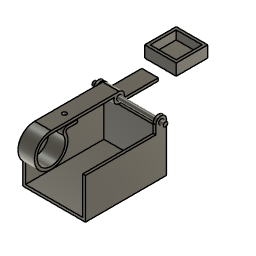
Card Holder v15 (Autodesk Fusion 360 design; units mm, degrees)
Autodesk Fusion 360 part; units mm, degrees
note: some values were not read from the file. Set by a fixed rule: which face or edge a step refers to.
sketch "Sketch1" plane through (0, 0, 0) normal (0, 0, 1) x (1, 0, 0)
  line L0 (0, 0) -> (66, 0)
  line L1 (66, 0) -> (66, 90.5)
  line L2 (66, 90.5) -> (0, 90.5)
  line L3 (0, 90.5) -> (0, 0)
  dimension "d12" = 66
  dimension "d13" = 90.5
  constraint horizontal L0
  constraint vertical L1
  constraint horizontal L2
  constraint vertical L3
  constraint coincident L0.start L3.end
  measures "d12" distance of L0.start L0.end
  measures "d13" distance of L0.end L1.end
extrude "Extrude1" add sketch "Sketch1" along normal blind 43.5 makes body 1
shell "Shell1" thickness 3.2 outward yes removed faces 2 at (44, 0, 14.5) at (22, 60.3333, 43.5) on bodies 1
sketch "Sketch2" plane through (-3.2, 0, 0) normal (-1, 0, 0) x (0, -1, 0)
  line L0 (-93.7, -3.2) -> (0, -3.2)
  line L1 (0, -3.2) -> (0, 43.5)
  line L2 (0, 43.5) -> (-93.7, 43.5)
  line L3 (-93.7, 43.5) -> (-93.7, -3.2)
  circle A0 centre (-87.6, 53.5) radius 2.5
  circle A1 centre (-87.6, 53.5) radius 2.9
  circle A2 centre (-87.6, 53.5) radius 6.1
  line L4 (-93.7, 53.5) -> (-93.7, 43.5)
  line L5 (-81.5, 53.5) -> (-81.5, 43.5)
  dimension "d17" = 5
  dimension "d18" = 0.4
  dimension "d19" = 3.2
  dimension "d20" = 10
  constraint concentric A0 A1
  constraint concentric A0 A2
  constraint coincident A2 L4.start
  constraint tangent A2 L4
  constraint coincident A2 L5.start
  constraint tangent A2 L5
  constraint vertical L4
  constraint vertical L5
  constraint horizontal L2.end L5.end
  constraint coincident L2.end L3.start
  measures "d17" diameter of A0
  measures "d18" distance of A0 A1
  measures "d19" distance of A1 A2
  measures "d20" distance of L2 A0.centre
extrude "Extrude2" add sketch "Sketch2" against normal up to surface (3.2 mm away) contours L2 A2 L4 L5 | A2 bodies 1
extrude "Extrude3" add sketch "Sketch2" against normal up to surface (3.2 mm away) from surface at -69.2 contours L2 A2 L4 L5 | A2 bodies 1
ref_plane "WorkPlane3" through (74.2, 46.85, 28.2) normal (1, 0, 0) x (0, 1, 0)
extrude "Extrude4" add sketch "Sketch2" along normal blind 5 and the other way up to surface (77.4 mm away) separate body contours A0 makes body 2
ref_plane "WorkPlane1" through (-3.2, 46.85, 28.2) normal (-1, 0, 0) x (0, -1, 0)
sketch "Sketch4" plane through (-3.2, 0, 0) normal (-1, 0, 0) x (0, -1, 0)
  circle A0 centre (-87.6, 53.5) radius 2.5
  circle A1 centre (-87.6, 53.5) radius 2.9
  circle A2 centre (-87.6, 53.5) radius 6.1
  line L0 (-87.6, 59.6) -> (2.9, 59.6)
  line L1 (2.9, 59.6) -> (2.9, 56.4)
  line L2 (2.9, 56.4) -> (-87.6, 56.4)
  line L3 (-32.7, 110) -> (-32.7, 124.9)
  line L4 (-32.7, 124.9) -> (-12.7, 124.9)
  line L5 (-12.7, 124.9) -> (-12.7, 110)
  line L6 (-32.7, 110) -> (-35.9, 110)
  line L7 (-35.9, 110) -> (-35.9, 128.1)
  line L8 (-35.9, 128.1) -> (-9.5, 128.1)
  line L9 (-9.5, 128.1) -> (-9.5, 110)
  line L10 (-12.7, 110) -> (-9.5, 110)
  line L11 (-87.6, 56.4) -> (-87.6, 59.6)
  circle A3 centre (-9, 40.225) radius 16.175
  circle A4 centre (-9, 40.225) radius 19.375
  line L12 (0, -3.2) -> (0, 43.5)
  line L13 (-39.575, 55.6) -> (-28.375, 55.6)
  line L14 (-28.375, 55.6) -> (-28.375, 52.4)
  line L15 (-28.375, 52.4) -> (-39.575, 52.4)
  line L16 (-39.575, 52.4) -> (-39.575, 55.6)
  circle A5 centre (-28.375, 50.0509) radius 2.3491
  circle A6 centre (-28.375, 50.0509) radius 5.5491
  line L17 (-132.85, 50.6) -> (-87.6, 50.6)
  line L18 (-87.6, 50.6) -> (-87.6, 47.4)
  line L19 (-87.6, 47.4) -> (-132.85, 47.4)
  line L20 (-132.85, 47.4) -> (-132.85, 50.6)
  dimension "d34" = 5.8
  dimension "d35" = 3.2
  dimension "d36" = 3.2
  dimension "d37" = 90.5
  dimension "d38" = 3.2
  dimension "d39" = 3.2
  dimension "d40" = 3.2
  dimension "d41" = 14.9
  dimension "d42" = 20
  dimension "d43" = 50.4
  dimension "d44" = 12.4
  dimension "d84" = 32.35
  dimension "d85" = 3.2
  dimension "d87" = 9
  dimension "d88" = 3.2
  dimension "d89" = 0.8
  dimension "d90" = 11.2
  dimension "d97" = 45.25
  dimension "d98" = 3.2
  constraint concentric A0 A1
  constraint concentric A0 A2
  constraint horizontal L0
  constraint vertical L1
  constraint horizontal L2
  constraint coincident A2 L0.start
  constraint vertical A0.centre L0.start
  constraint vertical L3
  constraint perpendicular L3 L4
  constraint perpendicular L4 L5
  constraint perpendicular L3 L6
  constraint perpendicular L6 L7
  constraint perpendicular L7 L8
  constraint perpendicular L8 L9
  constraint perpendicular L9 L10
  constraint horizontal L6.end L9.end
  constraint vertical L11
  constraint coincident L2.end L11.start
  constraint concentric A3 A4
  constraint tangent L0 A4
  constraint horizontal L13
  constraint vertical L14
  constraint horizontal L15
  constraint vertical L16
  constraint tangent A4 L14
  constraint concentric A5 A6
  constraint tangent A3 A6
  constraint tangent A4 A5
  constraint tangent L13 A6
  constraint coincident L14.end A5
  constraint horizontal L17
  constraint vertical L18
  constraint horizontal L19
  constraint vertical L20
  constraint collinear L11 L18
  constraint coincident A1 L17.end
  measures "d34" diameter of A1
  measures "d35" distance of A1 A2
  measures "d36" distance of L0.end L1.end
  measures "d37" distance of L0.start L0.end
  measures "d38" distance of L3.start L6.end
  measures "d39" distance of L5.end L9.end
  measures "d40" distance of L4 L8
  measures "d41" distance of L3.start L3.end
  measures "d42" distance of L3.end L4.end
  measures "d43" vertical distance of L0.end L9.end
  measures "d44" horizontal distance of L0.end L9.end
  measures "d84" diameter of A3
  measures "d85" distance of A3 A4
  measures "d87" distance of A3.centre L12
  measures "d88" distance of L13.start L15.end
  measures "d89" distance of L2 L13
  measures "d90" distance of L14.end L15.end
  measures "d97" distance of L18.end L19.end
  measures "d98" distance of L17.start L19.end
extrude "Extrude5" add sketch "Sketch4" against normal blind 19 from surface at -4.8 separate body contours A1 A2 L2 L18 | A2 L2 L11 | A1 A2 L11 L17 | A2 L17 L18 | A2 L0 L2 A4 | A2 L17 L19 L20 | L2 A4 | L2 A3 A4 L12 | A4 A6 | A4 L14 A5 A6 | A3 A4 L12 A6 | L13 L15 L16 A6 | L14 L15 A6 makes body 3
ref_plane "WorkPlane4" through (11.1, 48.3, 59.6) normal (0, 0, 1) x (0, -1, 0)
sketch "Sketch7" plane through (0, 0, 59.6) normal (0, 0, 1) x (1, 0, 0)
  line L0 (1.6, 39.575) -> (1.6, 28.375)
  line L1 (1.6, 28.375) -> (20.6, 28.375)
  line L2 (20.6, 28.375) -> (20.6, 39.575)
  line L3 (20.6, 39.575) -> (1.6, 39.575)
  circle A0 centre (11.1, 33.975) radius 2
  circle A1 centre (11.1, 33.975) radius 2.4
  point P0 (11.1, 39.575)
  dimension "d92" = 5.6
  dimension "d93" = 4
  dimension "d94" = 0.4
  constraint concentric A0 A1
  constraint midpoint L3 P0
  constraint vertical A0.centre P0
  measures "d92" distance of L3 A0.centre
  measures "d93" diameter of A0
  measures "d94" distance of A0 A1
extrude "Extrude10" cut sketch "Sketch7" against normal up to surface (7.2 mm away) contours A0 | A1 bodies 3
sketch "Sketch6" plane through (0, 0, 50.6) normal (0, 0, 1) x (-1, 0, 0)
  line L0 (-1.6, -87.6) -> (-1.6, -9)
  line L1 (-20.6, -9) -> (-20.6, -87.6)
  line L2 (3.9, -178.1) -> (-26.1, -178.1)
  line L3 (-26.1, -178.1) -> (-26.1, -148.1)
  line L4 (-26.1, -148.1) -> (3.9, -148.1)
  line L5 (3.9, -148.1) -> (3.9, -178.1)
  line L6 (7.1, -144.9) -> (7.1, -181.3)
  line L7 (7.1, -181.3) -> (-29.3, -181.3)
  line L8 (-29.3, -181.3) -> (-29.3, -144.9)
  line L9 (-29.3, -144.9) -> (7.1, -144.9)
  line L10 (-1.6, -9) -> (-20.6, -9)
  circle A0 centre (-11.1, -33.775) radius 2.4
  line L11 (-20.6, -87.6) -> (-1.6, -87.6)
  line L12 (-1.6, -132.85) -> (-1.6, -92.9666)
  line L13 (-1.6, -92.9666) -> (-20.6, -92.9666)
  line L14 (-20.6, -92.9666) -> (-20.6, -132.85)
  line L15 (-20.6, -132.85) -> (-1.6, -132.85)
  point P0 (-11.1, -178.1)
  point P1 (-11.1, -178.1)
  dimension "d76" = 30
  dimension "d77" = 30
  constraint horizontal L2
  constraint vertical L3
  constraint horizontal L4
  constraint vertical L5
  constraint midpoint L2 P1
  constraint coincident P1 P0
  measures "d76" distance of L2.start L2.end
  measures "d77" distance of L2.end L3.end
extrude "Extrude8" add sketch "Sketch6" along normal blind 3.2 separate body contours L2 L3 L4 L5 makes body 4
extrude "Extrude9" add sketch "Sketch6" along normal blind 13.2 contours L6 L7 L8 L9 bodies 4 3
ref_plane "WorkPlane2" through (11.1, 11.1, 110) normal (0, 0, -1) x (0, 1, 0)
sketch "Sketch5" plane through (0, 0, 110) normal (0, 0, -1) x (-1, 0, 0)
  circle A0 centre (-11.1, 41.5) radius 2
  circle A1 centre (-11.1, 41.5) radius 2.4
  line L0 (-1.6, 35.9) -> (-20.6, 35.9)
  circle A2 centre (-11.1, 3.9) radius 2
  circle A3 centre (-11.1, 3.9) radius 2.4
  line L1 (-1.6, 9.5) -> (-20.6, 9.5)
  line L2 (-1.6, 47.1) -> (-20.6, 47.1)
  line L3 (-20.6, 47.1) -> (-20.6, 35.9)
  line L4 (-20.6, 35.9) -> (-1.6, 35.9)
  line L5 (-1.6, 35.9) -> (-1.6, 47.1)
  line L6 (-1.6, -1.7) -> (-20.6, -1.7)
  line L7 (-20.6, -1.7) -> (-20.6, 9.5)
  line L8 (-20.6, 9.5) -> (-1.6, 9.5)
  line L9 (-1.6, 9.5) -> (-1.6, -1.7)
  point P0 (-11.1, 35.9)
  point P1 (-11.1, -1.7)
  point P2 (-11.1, 47.1)
  dimension "d49" = 4
  dimension "d51" = 0.4
  dimension "d53" = 4
  dimension "d55" = 0.4
  dimension "d67" = 5.6
  dimension "d68" = 5.6
  dimension "d70" = 5.6
  dimension "d71" = 5.6
  constraint concentric A0 A1
  constraint midpoint L0 P0
  constraint concentric A2 A3
  constraint vertical P0 A2.centre
  constraint horizontal L2
  constraint vertical L3
  constraint horizontal L4
  constraint vertical L5
  constraint coincident L0 L3.end
  constraint vertical L7
  constraint horizontal L8
  constraint vertical L9
  constraint coincident L1 L7.end
  constraint midpoint L6 P1
  constraint vertical A2.centre P1
  constraint horizontal L6
  constraint coincident L1.end L7.end
  constraint midpoint L2 P2
  constraint vertical A0.centre P2
  constraint coincident L0.start L4.end
  constraint vertical P0 A0.centre
  measures "d49" diameter of A0
  measures "d51" distance of A0 A1
  measures "d53" diameter of A2
  measures "d55" distance of A2 A3
  measures "d67" distance of A2.centre L8
  measures "d68" distance of A2.centre L6
  measures "d70" vertical distance of A0.centre P0
  measures "d71" distance of L2 A0.centre
extrude "Extrude6" [suppressed]
fillet "Fillet1" [suppressed]
extrude "Extrude7" [suppressed]
equation "CardWidth = 66 mm"
equation "CardHeight = 90.5 mm"
equation "CardDepth = 14.5 mm * 3"
equation "MotorHeight = 14.9 mm"
equation "MotorWidth = 20 mm"
equation "MotorPlatformDepth = 19 mm"
equation "Tolerance = 0.4 mm"
equation "RodDiameter = 5 mm"
equation "ScrewBigDiameter = 5.6 mm"
equation "ScrewSmallDiameter = 4 mm"
equation "WallThickness = 3.2 mm"
equation "d12 = CardWidth"
equation "d13 = CardHeight"
equation "d14 = CardDepth"
equation "d16 = WallThickness"
equation "d17 = RodDiameter"
equation "d18 = Tolerance"
equation "d19 = WallThickness"
equation "d34 = RodDiameter + 2 * Tolerance"
equation "d35 = WallThickness"
equation "d36 = WallThickness"
equation "d37 = CardHeight"
equation "d38 = WallThickness"
equation "d39 = WallThickness"
equation "d40 = WallThickness"
equation "d41 = MotorHeight"
equation "d42 = MotorWidth"
equation "d43 = Tolerance + 50 mm"
equation "d44 = 2 * WallThickness + ScrewSmallDiameter + 5 * Tolerance"
equation "d45 = -WallThickness - 4 * Tolerance"
equation "d46 = -MotorPlatformDepth"
equation "d49 = ScrewSmallDiameter"
equation "d51 = Tolerance"
equation "d53 = ScrewSmallDiameter"
equation "d55 = Tolerance"
equation "d57 = -WallThickness"
equation "d67 = WallThickness + ScrewSmallDiameter / 2 + Tolerance"
equation "d68 = d67"
equation "d70 = WallThickness + Tolerance + ScrewSmallDiameter / 2"
equation "d71 = d70"
equation "TrayWidth = 30 mm"
equation "TrayLength = 30 mm"
equation "TrayHeight = 10 mm"
equation "d76 = TrayWidth"
equation "d77 = TrayLength"
equation "d78 = -WallThickness"
equation "d79 = WallThickness"
equation "d81 = WallThickness + TrayHeight"
equation "MotorDiameter = 31.95 mm"
equation "d84 = MotorDiameter + Tolerance"
equation "d85 = WallThickness"
equation "d88 = WallThickness"
equation "d89 = Tolerance * 2"
equation "d90 = 2 * WallThickness + 2 * Tolerance + ScrewSmallDiameter"
equation "d92 = WallThickness + Tolerance + ScrewSmallDiameter / 2"
equation "d93 = ScrewSmallDiameter"
equation "d94 = Tolerance"
equation "d97 = CardHeight / 2"
equation "d98 = WallThickness"
